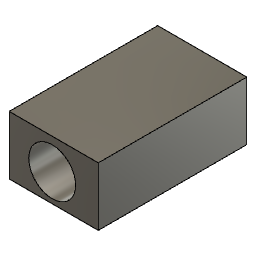
Lockwood tube FINAL DESIGN v1 v1 (Autodesk Fusion 360 design; units mm, degrees)
Autodesk Fusion 360 part; units mm, degrees
sketch "Sketch1" plane through (0, 0, 0) normal (0, 1, 0) x (1, 0, 0)
  line L0 (0, 0) -> (76.2, 0)
  line L1 (76.2, 0) -> (76.2, -203.2)
  line L2 (76.2, -203.2) -> (0, -203.2)
  line L3 (0, -203.2) -> (0, 0)
  dimension "d1" = 76.2
  dimension "d2" = 203.2
  constraint horizontal L0
  constraint vertical L1
  constraint horizontal L2
  constraint vertical L3
  constraint coincident L0.start L3.end
  measures "d1" distance of L0.start L0.end
  measures "d2" distance of L0.end L1.end
extrude "Extrude1" add sketch "Sketch1" along normal blind 50
hole "Hole1" at (36.7688, 23.7048, 203.2) direction (0, 0, -1) diameter 40 end through all
sketch "Sketch2" plane through (0, 50, 0) normal (0, 1, 0) x (-1, 0, 0)
  line L0 (0, 203.2) -> (-76.2, 203.2)
  line L1 (-76.2, 203.2) -> (-76.2, 0)
  line L2 (-76.2, 0) -> (0, 0)
  line L3 (0, 0) -> (0, 203.2)
  line L4 (150, 0) -> (73.8, 0)
  line L5 (73.8, 0) -> (73.8, 127)
  line L6 (73.8, 127) -> (150, 127)
  line L7 (150, 127) -> (150, 0)
  dimension "d8" = 76.2
  dimension "d9" = 127
  constraint horizontal L4
  constraint vertical L5
  constraint horizontal L6
  constraint vertical L7
  measures "d8" distance of L4.start L4.end
  measures "d9" distance of L4.start L6.end
sketch "Sketch3" plane through (0, 0, 0) normal (0, 1, 0) x (1, 0, 0)
  line L0 (79.4367, 34.7313) -> (3.2367, 34.7313)
  line L1 (3.2367, 34.7313) -> (3.2367, 237.9313)
  line L2 (3.2367, 237.9313) -> (79.4367, 237.9313)
  line L3 (79.4367, 237.9313) -> (79.4367, 34.7313)
  dimension "d13" = 76.2
  dimension "d14" = 203.2
  constraint horizontal L0
  constraint vertical L1
  constraint horizontal L2
  constraint vertical L3
  measures "d13" distance of L0.start L0.end
  measures "d14" distance of L0.start L2.end
move_face "OffsetFaces1" offset -76.2 1 faces at (69.7043, 25.0665, 203.2)
